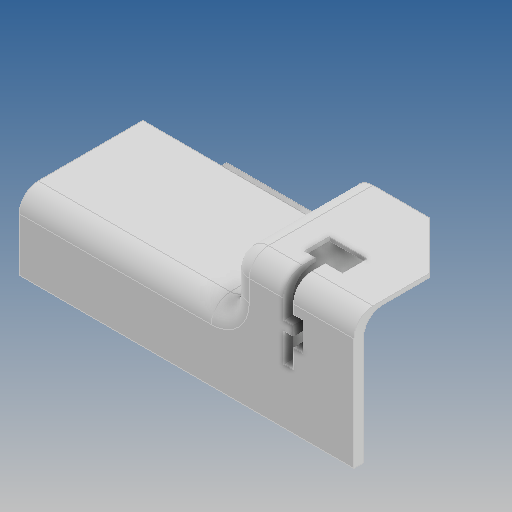
# Autodesk Inventor part: 0008-30-011
Saved by Autodesk Inventor 2020 (Build 240168000, 168)
## iProperties
Created: 2021-05-29
Part Number: 0008-30-011
Material: Generic
Document SubType Name: Modeling
Designer: Iulian Bors
Density: 1 g/cm^3
Appearance: Default
Author: Iulian Bors
Subject: 011
Autodesk Inventor part; units mm, degrees
ref_plane "YZ Plane" through (0, 0, 0) normal (1, 0, 0) x (0, 1, 0)
ref_plane "XZ Plane" through (0, 0, 0) normal (0, 1, 0) x (-1, 0, 0)
ref_plane "XY Plane" through (0, 0, 0) normal (0, 0, 1) x (1, 0, 0)
sketch "Sketch1" plane through (0, 0, 0) normal (0, 0, 1) x (1, 0, 0)
  line L0 (-88.5, 34.5) -> (88.5, 34.5)
  line L1 (88.5, 34.5) -> (88.5, -34.5)
  line L2 (88.5, -34.5) -> (-88.5, -34.5)
  line L3 (-88.5, -34.5) -> (-88.5, 34.5)
  point P0 (0, 0)
  point P1 (-88.5, 0)
  point P2 (0, 34.5)
  dimension "d0" = 177
  dimension "d1" = 69
  constraints: 8 end point, 2 midpoint, 2 parallel, 1 horizontal, 1 horizontal alignment, 1 perpendicular, 1 vertical alignment
  measures "d0" distance of L0.start L0.end
  measures "d1" distance of L2.end L0.start
sketch "Sketch1 outline for Extrusion1" plane through (0, 0, 0) normal (0, 0, 1) x (1, 0, 0)
  line L0 (-88.5, -34.5) -> (88.5, -34.5)
  line L1 (-88.5, 34.5) -> (-88.5, -34.5)
  line L2 (88.5, 34.5) -> (-88.5, 34.5)
  line L3 (88.5, -34.5) -> (88.5, 34.5)
extrude "Extrusion1" add sketch "Sketch1 outline for Extrusion1" along normal blind 65
sketch "Sketch2" plane through (0, 0, 0) normal (0, 0, -1) x (-1, 0, 0)
  line L0 (232.5, 3.5) -> (-12.5, 3.5) projected
  line L1 (88.5, 34.5) -> (88.5, -34.5) projected
  line L2 (-88.5, 34.5) -> (88.5, 34.5) projected
  line L3 (-22.5, 34.5) -> (-22.5, 3.5)
  line L4 (-22.5, 13.5) -> (-22.5, 24.5) projected
  line L5 (-12.5, 3.5) -> (-22.5, 3.5)
  point P0 (0, 0)
  point P1 (88.5, 3.5)
  constraints: 4 end point, 1 collinear, 1 horizontal, 1 vertical, 2 other
sketch "Sketch2 outline for Extrusion2" plane through (0, 0, 0) normal (0, 0, -1) x (-1, 0, 0)
  line L0 (-22.5, 3.5) -> (-12.5, 3.5)
  line L1 (-22.5, 34.5) -> (-22.5, 3.5)
  line L2 (88.5, 34.5) -> (-22.5, 34.5)
  line L3 (88.5, 3.5) -> (88.5, 34.5)
  line L4 (-12.5, 3.5) -> (88.5, 3.5)
extrude "Extrusion2" cut sketch "Sketch2 outline for Extrusion2" against normal through all
fillet "Fillet1" radius 10 2 edges at (22.5, 3.5, 32.5) (22.5, 34.5, 32.5)
sketch "Sketch3" plane through (0, 0, 0) normal (0, 0, -1) x (-1, 0, 0)
  line L0 (-43.5, -11.5) -> (216.5, -11.5) projected
  line L1 (-43.5, 32.5) -> (-43.5, -11.5) projected
  line L2 (-90.5, 32.5) -> (-43.5, 32.5) projected
  line L3 (-88.5, 32.5) -> (-88.5, -34.5)
  line L4 (-88.5, -34.5) -> (88.5, -34.5)
  line L5 (88.5, -34.5) -> (88.5, -11.5)
  line L6 (88.5, 3.5) -> (88.5, -34.5) projected
  line L7 (88.5, -34.5) -> (-88.5, -34.5) projected
  line L8 (-88.5, -34.5) -> (-88.5, 34.5) projected
  point P0 (0, 0)
  constraints: 6 end point, 3 collinear, 2 point on line
sketch "Sketch3 outline for Extrusion3" plane through (0, 0, 0) normal (0, 0, -1) x (-1, 0, 0)
  line L0 (-43.5, -11.5) -> (-43.5, 32.5)
  line L1 (88.5, -11.5) -> (-43.5, -11.5)
  line L2 (88.5, -34.5) -> (88.5, -11.5)
  line L3 (-88.5, -34.5) -> (88.5, -34.5)
  line L4 (-88.5, 32.5) -> (-88.5, -34.5)
  line L5 (-43.5, 32.5) -> (-88.5, 32.5)
extrude "Extrusion3" cut sketch "Sketch3 outline for Extrusion3" against normal blind 60
sketch "Sketch4" plane through (88.5, 34.5, 65) normal (0, 1, 0) x (1, 0, 0)
  line L0 (0, 65) -> (-56, 65)
  line L1 (0, 65) -> (0, 0)
  line L2 (0, 40) -> (-25, 65)
  line L3 (0, 38.585786) -> (-26.414214, 65)
  point P0 (-88.5, 65)
  dimension "d40" = 1
  constraints: 2 end point, 2 point on line, 1 parallel
  measures "d40" distance between parallel lines of L2 L3
sketch "Sketch4 outline for Extrusion4" plane through (88.5, 34.5, 65) normal (0, 1, 0) x (1, 0, 0)
  line L0 (0, 65) -> (-26.414214, 65)
  line L1 (-26.414214, 65) -> (0, 38.585786)
  line L2 (0, 38.585786) -> (0, 65)
extrude "Extrusion4" cut sketch "Sketch4 outline for Extrusion4" against normal blind 60
sketch "Sketch5" plane through (0, 0, 65) normal (0, 0, 1) x (1, 0, 0)
  line L0 (50.5, -5.5) -> (55.5, -5.5)
  line L1 (55.5, -5.5) -> (55.5, 9.5)
  line L2 (55.5, 9.5) -> (50.5, 9.5)
  line L3 (50.5, 9.5) -> (50.5, -5.5)
  line L4 (-88.5, -34.5) -> (88.5, -34.5) projected
  line L5 (88.5, -34.5) -> (88.5, 34.5) projected
  line L6 (55.5, 9.5) -> (60.5, 9.5)
  line L7 (60.5, 9.5) -> (60.5, 4.5)
  line L8 (60.5, 4.5) -> (55.5, 4.5)
  line L9 (55.5, 4.5) -> (55.5, 9.5)
  line L10 (55.5, 19.5) -> (60.5, 19.5)
  line L11 (60.5, 19.5) -> (60.5, 9.5)
  line L12 (60.5, 9.5) -> (55.5, 9.5)
  line L13 (55.5, 9.5) -> (55.5, 19.5)
  line L14 (50.5, 19.5) -> (55.5, 19.5)
  line L15 (55.5, 19.5) -> (55.5, 14.5)
  line L16 (55.5, 14.5) -> (50.5, 14.5)
  line L17 (50.5, 14.5) -> (50.5, 19.5)
  line L18 (50.5, 34.5) -> (55.5, 34.5)
  line L19 (55.5, 34.5) -> (55.5, 19.5)
  line L20 (55.5, 19.5) -> (50.5, 19.5)
  line L21 (50.5, 19.5) -> (50.5, 34.5)
  line L22 (88.5, 34.5) -> (32.5, 34.5) projected
  point P0 (0, 0)
  dimension "d11" = 5
  dimension "d13" = 33
  dimension "d20" = 5
  dimension "d21" = 10
  dimension "d23" = 15
  dimension "d24" = 15
  constraints: 40 end point, 11 parallel, 10 collinear, 6 perpendicular, 4 horizontal
  measures "d11" distance of L1.end L2.end
  measures "d13" distance between parallel lines of L5 L1
  measures "d20" distance of L7.end L8.end
  measures "d21" distance of L10.end L11.end
  measures "d23" distance of L2.end L0.start
  measures "d24" distance of L20.end L18.start
sketch "Sketch5 outline for Extrusion5" plane through (0, 0, 65) normal (0, 0, 1) x (1, 0, 0)
  line L0 (55.5, 9.5) -> (50.5, 9.5)
  line L1 (50.5, 9.5) -> (50.5, -5.5)
  line L2 (50.5, -5.5) -> (55.5, -5.5)
  line L3 (55.5, -5.5) -> (55.5, 4.5)
  line L4 (55.5, 4.5) -> (60.5, 4.5)
  line L5 (60.5, 4.5) -> (60.5, 19.5)
  line L6 (60.5, 19.5) -> (55.5, 19.5)
  line L7 (55.5, 19.5) -> (55.5, 34.5)
  line L8 (55.5, 34.5) -> (50.5, 34.5)
  line L9 (50.5, 34.5) -> (50.5, 14.5)
  line L10 (50.5, 14.5) -> (55.5, 14.5)
  line L11 (55.5, 14.5) -> (55.5, 9.5)
extrude "Extrusion5" cut sketch "Sketch5 outline for Extrusion5" against normal blind 30
sketch "Sketch6" plane through (0, 0, 0) normal (0, 0, -1) x (-1, 0, 0)
  line L0 (-28.5, 18.5) -> (-33.5, 18.5) projected
  line L1 (-33.5, 18.5) -> (-33.5, 8.5) projected
  line L2 (-28.5, 8.5) -> (-28.5, 18.5) projected
  line L3 (-33.5, 8.5) -> (-28.5, 8.5) projected
  line L4 (54.5, -1.5) -> (4.5, -1.5) projected
  line L5 (4.5, -1.5) -> (4.5, -6.5) projected
  line L6 (4.5, -6.5) -> (54.5, -6.5) projected
  line L7 (54.5, -6.5) -> (54.5, -1.5) projected
  line L8 (4.65, -1.65) -> (54.35, -1.65)
  line L9 (54.35, -1.65) -> (54.35, -6.35)
  line L10 (54.35, -6.35) -> (4.65, -6.35)
  line L11 (4.65, -6.35) -> (4.65, -1.65)
  line L12 (-33.35, 8.65) -> (-33.35, 18.35)
  line L13 (-33.35, 18.35) -> (-28.65, 18.35)
  line L14 (-28.65, 18.35) -> (-28.65, 8.65)
  line L15 (-28.65, 8.65) -> (-33.35, 8.65)
  line L16 (-33.35, 16.85) -> (-28.65, 16.85)
  line L17 (-33.35, 10.15) -> (-28.65, 10.15)
  line L18 (6.65, -6.35) -> (6.65, -1.65)
  line L19 (52.35, -6.35) -> (52.35, -1.65)
  point P0 (0, 0)
  dimension "d17" = 0.15
  dimension "d35" = 0.15
  dimension "d36" = 1.5
  dimension "d37" = 1.5
  dimension "d38" = 2
  dimension "d39" = 2
  constraints: 24 end point, 8 point on line, 3 perpendicular, 1 parallel, 6 other
  measures "d17" distance between parallel lines of L4 L8
  measures "d35" distance between parallel lines of L12 L1
  measures "d36" distance between parallel lines of L15 L17
  measures "d37" distance between parallel lines of L13 L16
  measures "d38" distance between parallel lines of L9 L19
  measures "d39" distance between parallel lines of L18 L11
sketch "Sketch6 outline for Extrusion6" plane through (0, 0, 0) normal (0, 0, -1) x (-1, 0, 0)
  line L0 (-33.35, 10.15) -> (-28.65, 10.15)
  line L1 (-33.35, 16.85) -> (-33.35, 10.15)
  line L2 (-28.65, 16.85) -> (-33.35, 16.85)
  line L3 (-28.65, 10.15) -> (-28.65, 16.85)
  line L4 (52.35, -6.35) -> (52.35, -1.65)
  line L5 (6.65, -6.35) -> (52.35, -6.35)
  line L6 (6.65, -1.65) -> (6.65, -6.35)
  line L7 (52.35, -1.65) -> (6.65, -1.65)
extrude "Extrusion6" add sketch "Sketch6 outline for Extrusion6" along normal blind 8
fillet "Fillet2" radius 10 6 edges at (72, 34.5, 65) (25.4289, 31.5711, 65) (22.5, 19, 65) (19.5711, 6.4289, 65) (-38, 3.5, 65) (41.5, 34.5, 65)
sketch "Sketch7" plane through (32.5, 34.5, 0) normal (0, 1, 0) x (1, 0, 0)
  line L0 (32, -48) -> (12, -48)
  line L1 (12, -48) -> (12, -35)
  line L2 (12, -35) -> (32, -35)
  line L3 (32, -35) -> (32, -48)
  line L4 (18, -35) -> (23, -35) projected
  point P0 (-32.5, 0)
  point P1 (20.5, -35)
  dimension "d26" = 20
  dimension "d27" = 13
  constraints: 8 end point, 2 parallel, 1 collinear, 1 horizontal, 1 midpoint, 1 perpendicular
  measures "d26" distance of L1.end L2.end
  measures "d27" distance of L2.end L0.start
sketch "Sketch7 outline for Extrusion7" plane through (32.5, 34.5, 0) normal (0, 1, 0) x (1, 0, 0)
  line L0 (12, -35) -> (12, -48)
  line L1 (32, -35) -> (12, -35)
  line L2 (32, -48) -> (32, -35)
  line L3 (12, -48) -> (32, -48)
extrude "Extrusion7" cut sketch "Sketch7 outline for Extrusion7" against normal blind 30
move faces "Move1" translate (-1, 0, 0) faces at (88.5, 7.5, 61.666667)
fillet "Fillet3" radius 10 2 edges at (71.5, 32.5, 60) (47, 32.5, 60)
body "Solid1"
